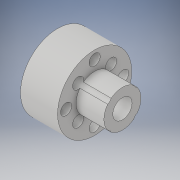
# Autodesk Inventor part: WheelandSprocketComboHub
Saved by Autodesk Inventor 2017 (Build 210142000, 142)
## iProperties
Created: 2018-04-04
Part Number: WheelandSprocketComboHub
Material: Generic
Document SubType Name: Modeling
Designer: User
Density: 1 g/cm^3
Appearance: Default
Author: User
Autodesk Inventor part; units mm, degrees
ref_plane "YZ Plane" through (0, 0, 0) normal (1, 0, 0) x (0, 1, 0)
ref_plane "XZ Plane" through (0, 0, 0) normal (0, 1, 0) x (-1, 0, 0)
ref_plane "XY Plane" through (0, 0, 0) normal (0, 0, 1) x (1, 0, 0)
sketch "Sketch1" plane through (0, 0, 0) normal (1, 0, 0) x (0, 1, 0)
  circle A0 centre (0, 0) radius 12.7
  line L0 (5.6576, -5.6576) -> (0, 0)
  line L1 (0, 0.0631) -> (0, -4.7425)
  circle A1 centre (0, 0) radius 3.302
  point P0 (5.6576, 5.6576)
  point P1 (-5.6576, 5.6576)
  point P2 (-5.6576, -5.6576)
  point P3 (9.779, 0)
  point P4 (0, 9.779)
  point P5 (-9.779, 0)
  point P6 (0, -9.779)
  point P7 (5.6576, 5.6576)
  point P8 (-5.6576, 5.6576)
  point P9 (-5.6576, -5.6576)
  dimension "d0" = 25.4
  dimension "d6" = 45
  dimension "d15" = 6.604
  dimension "d23" = 360
  dimension "d25" = 9.779
  dimension "d28" = 360
  constraints: 5 coincident, 4 end point, 2 centre point, 2 point on line, 1 vertical, 10 other
  measures "d0" diameter of A0
  measures "d6" angle of L1 L0
  measures "d15" diameter of A1
  measures "d25" distance of point (0, 0) point (9.779, 0)
extrude "Extrusion1" add sketch "Sketch1" along normal blind 12.7
sketch "Sketch2" plane through (12.7, 0, 0) normal (1, 0, 0) x (0, 0, -1)
  circle A0 centre (0, 0) radius 3.302 projected
  circle A1 centre (0, 0) radius 6.35
  point P0 (0, 0)
  dimension "d18" = 12.7
  constraints: 1 centre point, 1 coincident
  measures "d18" diameter of A1
extrude "Extrusion2" add sketch "Sketch2" along normal blind 9.525
hole "Hole1" at (0, 9.779, 0) at (0, 0, 9.779) at (0, -9.779, 0) at (0, 0, -9.779) direction (1, 0, 0) diameter 3.81 end through all
hole "Hole2" at (0, 5.6576, 5.6576) at (0, -5.6576, 5.6576) at (0, -5.6576, -5.6576) at (0, 5.6576, -5.6576) direction (1, 0, 0) diameter 3.81 end through all
body "Solid1"
